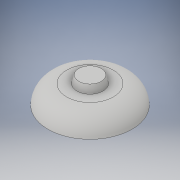
# Autodesk Inventor part: cup
Saved by Autodesk Inventor 2019.3 (Build 233278000, 278)
## iProperties
Created: 2019-04-14
Part Number: cup
Material: Generic
Document SubType Name: Modeling
Designer: peter
Density: 1 g/cm^3
Appearance: Default
Author: peter
Autodesk Inventor part; units mm, degrees
note: some values were not read from the file. Chosen so that the rebuilt part matches the saved one: side of "Thicken1".
ref_plane "YZ Plane" through (0, 0, 0) normal (1, 0, 0) x (0, 1, 0)
ref_plane "XZ Plane" through (0, 0, 0) normal (0, 1, 0) x (-1, 0, 0)
ref_plane "XY Plane" through (0, 0, 0) normal (0, 0, 1) x (1, 0, 0)
sketch "Sketch1" plane through (0, 0, 0) normal (0, 0, 1) x (1, 0, 0)
  line L0 (0, 0) -> (22.5, 0) construction
  line L1 (0, 0) -> (0, 10) construction
  line L2 (0, 10) -> (7, 10) construction
  line L3 (7, 10) -> (0, 10) construction
  line L4 (0, 10) -> (0, 14) construction
  line L5 (0, 14) -> (6, 14) construction
  line L6 (0, 10) -> (12.5, 10) construction
  line L7 (6, 14) -> (7, 10)
  line L8 (7, 10) -> (12.5, 10)
  line L9 (12.5, 10) -> (12.5, 10)
  line L10 (22.5, 0) -> (22.5, 0)
  arc A0 (22.5, 0) -> (12.5, 10) centre (12.5, 0) ccw
  line L11 (6, 14) -> (0, 14)
  point P0 (22.5, 10)
  dimension "d0" = 22.5
  dimension "d1" = 10
  dimension "d2" = 7
  dimension "d3" = 4
  dimension "d4" = 6
  dimension "d5" = 12.5
  dimension "d6" = 10
  constraints: 24 end point, 4 point on line, 3 horizontal, 3 perpendicular, 2 point on circle, 2 tangent, 2 vertical, 1 centre point, 1 collinear
  measures "d0" distance of L0.start L0.end
  measures "d1" distance of L0.start L1.end
  measures "d2" distance of L1.end L2.end
  measures "d3" distance of L1.end L4.end
  measures "d4" distance of L4.end L5.end
  measures "d5" distance of L1.end L6.end
  measures "d6" radius of A0
surface revolve "RevolutionSrf1" sketch "Sketch1" angle 360 about axis through (0, 0, 0) along (0, 1, 0) shown no curves L10 A0 L9 L8 L7 L11
thicken "Thicken1" operation new thickness 2 both sides no extend neighbours no toward (0, -1, 0) faces at (-0.7092, 14, -1.4219) (6.4729, 11.3333, 1.5954) (10.5456, 10, 0.9971) (22.181, 0.7473, 3.6048)
body "Solid1"
body "Srf1"
